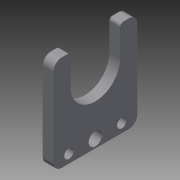
# Autodesk Inventor part: motor mount
Saved by Autodesk Inventor 2015 SP1 (Build 190203100, 203)
## iProperties
Created: 2016-07-07
Part Number: motor mount
Material: Generic
Document SubType Name: Modeling
Designer: lustinga
Density: 1 g/cm^3
Appearance: Default
Mass: 10.8386 g
Surface Area: 85.0658 cm^2
Volume: 10.8386 cm^3
Author: lustinga
Autodesk Inventor part; units mm, degrees
ref_plane "YZ Plane" through (0, 0, 0) normal (1, 0, 0) x (0, 1, 0)
ref_plane "XZ Plane" through (0, 0, 0) normal (0, 1, 0) x (-1, 0, 0)
ref_plane "XY Plane" through (0, 0, 0) normal (0, 0, 1) x (1, 0, 0)
sketch "Sketch1" plane through (0, 0, 0) normal (1, 0, 0) x (0, 1, 0)
  arc A0 (1.0277, 65.9115) -> (30.5255, 66.0516) centre (15.7774, 65.8167) ccw
  line L0 (30.5255, 66.0516) -> (30.5255, 81.9568)
  line L1 (40.7755, 78.9568) -> (40.7755, 31.8167)
  circle A1 centre (15.7774, 31.8167) radius 4
  line L2 (-9.2226, 78.8167) -> (-9.2226, 31.8167)
  line L3 (1.0277, 65.9115) -> (1.0277, 81.8167)
  line L4 (-4.2226, 83.8167) -> (-0.9723, 83.8167)
  line L5 (32.5255, 83.9568) -> (35.7755, 83.9568)
  circle A2 centre (0.0401, 32.0007) radius 2.8
  circle A3 centre (31.5401, 32.0007) radius 2.8
  line L6 (15.7774, 31.8167) -> (15.7774, 44.8985) construction
  arc A4 (40.7755, 78.9568) -> (35.7755, 83.9568) centre (35.7755, 78.9568) ccw
  arc A5 (-4.2226, 83.8167) -> (-9.2226, 78.8167) centre (-4.2226, 78.8167) ccw
  line L7 (-4.2226, 26.8167) -> (35.7755, 26.8167)
  arc A6 (-9.2226, 31.8167) -> (-4.2226, 26.8167) centre (-4.2226, 31.8167) ccw
  arc A7 (35.7755, 26.8167) -> (40.7755, 31.8167) centre (35.7755, 31.8167) ccw
  arc A8 (32.5255, 83.9568) -> (30.5255, 81.9568) centre (32.5255, 81.9568) ccw
  arc A9 (1.0277, 81.8167) -> (-0.9723, 83.8167) centre (-0.9723, 81.8167) ccw
  point P0 (-9.2226, 83.8167)
  point P1 (30.5255, 83.9568)
  point P2 (40.7755, 83.9568)
  point P3 (1.0277, 83.8167)
  dimension "d21" = 29.5
  dimension "d44" = 8
  dimension "d57" = 25
  dimension "d64" = 5.6
  dimension "d74" = 18
  dimension "d76" = 5
  dimension "d79" = 2
  constraints: 16 end point, 14 point on circle, 12 tangent, 10 centre point, 8 point on line, 3 equal radius, 3 vertical, 2 horizontal, 1 coincident, 1 parallel, 1 vertical alignment, 1 other
  measures "d21" diameter of A0
  measures "d44" diameter of A1
  measures "d57" distance from line of L2 A0.centre
  measures "d64" diameter of A3
  measures "d74" distance from line of L4 A0.centre
  measures "d76" radius of A4
  measures "d79" radius of A8
extrude "Extrusion2" add sketch "Sketch1" along normal blind 6.35
body "Solid2"
